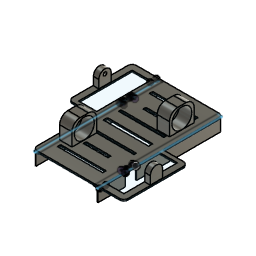
Chassis V4 (Autodesk Fusion 360 design; units mm, degrees)
Autodesk Fusion 360 part; units mm, degrees
note: some values were not read from the file. Set by a fixed rule: which sketch regions a step uses.
sketch "Sketch1" plane through (0, 0, 0) normal (0, 0, 1) x (1, 0, 0)
  line L0 (0, 0) -> (140, 0)
  line L1 (140, 0) -> (140, 150)
  line L2 (140, 150) -> (0, 150)
  line L3 (0, 150) -> (0, 0)
  dimension "d1" = 140
  dimension "d2" = 150
  constraint horizontal L0
  constraint vertical L1
  constraint horizontal L2
  constraint vertical L3
  constraint coincident L0.start L3.end
  measures "d1" distance of L0.start L0.end
  measures "d2" distance of L0.start L2.end
extrude "Extrude1" add sketch "Sketch1" along normal blind 1.75 makes body 1
sketch "Sketch2" plane through (0, 0, 1.75) normal (0, 0, 1) x (-1, 0, 0)
  line L0 (0, -150) -> (0, 0)
  line L1 (0, 0) -> (-140, 0)
  line L2 (-140, 0) -> (-140, -150)
  line L3 (-140, -150) -> (0, -150)
  line L4 (-7.5, -7.5) -> (-132.5, -7.5)
  line L5 (-132.5, -7.5) -> (-132.5, -142.5)
  line L6 (-132.5, -142.5) -> (-7.5, -142.5)
  line L7 (-7.5, -142.5) -> (-7.5, -7.5)
  line L8 (-7.5, -142.5) -> (-29.5, -142.5)
  line L9 (-29.5, -142.5) -> (-29.5, -77.5)
  line L10 (-29.5, -77.5) -> (-7.5, -77.5)
  line L11 (-7.5, -77.5) -> (-7.5, -142.5)
  line L12 (-132.5, -142.5) -> (-132.5, -77.5)
  line L13 (-110.5, -142.5) -> (-132.5, -142.5)
  line L14 (-132.5, -77.5) -> (-110.5, -77.5)
  line L15 (-110.5, -77.5) -> (-110.5, -142.5)
  line L16 (-29.5, -72.5) -> (-29.5, -7.5)
  line L17 (-7.5, -72.5) -> (-29.5, -72.5)
  line L18 (-29.5, -7.5) -> (-7.5, -7.5)
  line L19 (-7.5, -7.5) -> (-7.5, -72.5)
  line L20 (-132.5, -72.5) -> (-132.5, -7.5)
  line L21 (-110.5, -72.5) -> (-132.5, -72.5)
  line L22 (-132.5, -7.5) -> (-110.5, -7.5)
  line L23 (-110.5, -7.5) -> (-110.5, -72.5)
  dimension "d5" = -7.5
  dimension "d6" = 22
  dimension "d7" = 65
  dimension "d10" = -103
  dimension "d11" = 70
  constraint horizontal L8
  constraint vertical L9
  constraint horizontal L10
  constraint vertical L11
  measures "d6" distance of L6.end L8.end
  measures "d7" distance of L6.end L10.end
extrude "Extrude2" cut sketch "Sketch2" against normal up to surface (1.75 mm away) contours L4 L7 L16 L17 L18 L19 | L4 L5 L20 L21 L22 L23 | L6 L7 L8 L9 L10 L11 | L5 L6 L12 L13 L14 L15 bodies 1
sketch "Sketch3" plane through (0, 0, 1.75) normal (0, 0, 1) x (-1, 0, 0)
  line L0 (-110.5, -7.5) -> (-110.5, -72.5)
  line L1 (-132.5, -72.5) -> (-132.5, -7.5)
  line L2 (-132.5, -7.5) -> (-110.5, -7.5)
  line L3 (-110.5, -77.5) -> (-110.5, -142.5)
  line L4 (-110.5, -142.5) -> (-132.5, -142.5)
  line L5 (-132.5, -142.5) -> (-132.5, -77.5)
  line L6 (-132.5, -77.5) -> (-110.5, -77.5)
  line L7 (-7.5, -77.5) -> (-7.5, -142.5)
  line L8 (-7.5, -142.5) -> (-29.5, -142.5)
  line L9 (-29.5, -142.5) -> (-29.5, -77.5)
  line L10 (-29.5, -77.5) -> (-7.5, -77.5)
  line L11 (-7.5, -7.5) -> (-7.5, -72.5)
  line L12 (-29.5, -72.5) -> (-29.5, -7.5)
  line L13 (-29.5, -7.5) -> (-7.5, -7.5)
  line L14 (0, -150) -> (0, 0)
  line L15 (0, 0) -> (-140, 0)
  line L16 (-140, 0) -> (-140, -150)
  line L17 (-140, -150) -> (0, -150)
  line L18 (-29.5, -110) -> (-110.5, -110) construction
  line L19 (-29.5, -40) -> (-110.5, -40) construction
  line L20 (-29.5, -110) -> (-33.25, -110) construction
  line L21 (-30.0705, -117.5) -> (-36.4295, -117.5)
  line L22 (-36.4295, -117.5) -> (-36.4295, -102.5)
  line L23 (-36.4295, -102.5) -> (-30.0705, -102.5)
  line L24 (-30.0705, -102.5) -> (-30.0705, -117.5)
  line L25 (-30.0705, -117.5) -> (-36.4295, -102.5) construction
  line L26 (-36.4295, -117.5) -> (-30.0705, -102.5) construction
  line L27 (-103.5705, -47.5) -> (-109.9295, -47.5)
  line L28 (-103.5705, -32.5) -> (-103.5705, -47.5)
  line L29 (-109.9295, -32.5) -> (-103.5705, -32.5)
  line L30 (-109.9295, -47.5) -> (-109.9295, -32.5)
  line L31 (-110.5, -110) -> (-140, -110) construction
  line L32 (-33.25, -117.5) -> (-33.25, -110) construction
  line L33 (-33.25, -110) -> (-33.25, -102.5) construction
  circle A0 centre (-33.25, -113.75) radius 1.5
  circle A1 centre (-33.25, -106.25) radius 1.5
  line L34 (-106.75, -47.5) -> (-106.75, -40) construction
  line L35 (-106.75, -40) -> (-106.75, -32.5) construction
  circle A2 centre (-106.75, -43.75) radius 1.5
  circle A3 centre (-106.75, -36.25) radius 1.5
  line L36 (-7.5, -110) -> (0, -110) construction
  line L37 (-7.0568, -117.5) -> (-0.4432, -117.5)
  line L38 (-0.4432, -117.5) -> (-0.4432, -102.5)
  line L39 (-0.4432, -102.5) -> (-7.0568, -102.5)
  line L40 (-7.0568, -102.5) -> (-7.0568, -117.5)
  line L41 (-7.0568, -117.5) -> (-0.4432, -102.5) construction
  line L42 (-0.4432, -117.5) -> (-7.0568, -102.5) construction
  line L43 (-139.5568, -47.5) -> (-132.9432, -47.5)
  line L44 (-139.5568, -32.5) -> (-139.5568, -47.5)
  line L45 (-132.9432, -32.5) -> (-139.5568, -32.5)
  line L46 (-132.9432, -47.5) -> (-132.9432, -32.5)
  line L47 (-110.5, -72.5) -> (-132.5, -72.5)
  line L48 (-7.5, -72.5) -> (-29.5, -72.5)
  point P0 (-33.25, -110)
  point P1 (-3.75, -110)
  dimension "d14" = 3.75
  dimension "d15" = 15
  dimension "d18" = -73.5
  dimension "d19" = 70
  dimension "d26" = 3
  dimension "d27" = 3
  dimension "d28" = 3
  dimension "d29" = 3
  dimension "d49" = 15
  dimension "d52" = -132.5
  dimension "d53" = 70
  constraint midpoint L9 L18.start
  constraint midpoint L3 L18.end
  constraint midpoint L12 L19.start
  constraint midpoint L0 L19.end
  constraint perpendicular L9 L20
  constraint horizontal L21
  constraint perpendicular L21 L22
  constraint parallel L21 L23
  constraint parallel L22 L24
  constraint coincident L25 P0
  constraint coincident L26 P0
  constraint coincident P0 L20.end
  constraint coincident L16 L31.end
  constraint perpendicular L16 L31
  constraint midpoint L21 L32.start
  constraint midpoint L23 L33.end
  constraint midpoint L32 A0.centre
  constraint midpoint L33 A1.centre
  constraint midpoint L27 L34.start
  constraint coincident L19 L34.end
  constraint perpendicular L19 L34
  constraint midpoint L29 L35.end
  constraint midpoint L34 A2.centre
  constraint midpoint L35 A3.centre
  constraint midpoint L7 L36.start
  constraint coincident L14 L36.end
  constraint perpendicular L14 L36
  constraint horizontal L37
  constraint perpendicular L37 L38
  constraint parallel L37 L39
  constraint parallel L38 L40
  constraint coincident L41 P1
  constraint coincident L42 P1
  constraint midpoint L36 P1
  measures "d14" distance of L18.start P0
  measures "d15" distance of L21.end L22.end
  measures "d26" diameter of A0
  measures "d27" diameter of A1
  measures "d28" diameter of A2
  measures "d29" diameter of A3
  measures "d49" distance of L37.end L38.end
extrude "Extrude3" add sketch "Sketch3" along normal blind 17.5 contours L37 L38 L39 L40 | L43 L44 L45 L46 bodies 1
extrude "Extrude4" cut sketch "Sketch3" against normal up to surface (1.75 mm away) contours A0 | A1 | A2 | A3 bodies 1
sketch "Sketch4" plane through (132.5, 0, 0) normal (-1, 0, 0) x (0, -1, 0)
  line L0 (-72.5, 0) -> (-7.5, 0)
  line L1 (-7.5, 0) -> (-7.5, 1.75)
  line L2 (-72.5, 1.75) -> (-7.5, 1.75) construction
  line L3 (-40, 1.75) -> (-40, 13.875) construction
  circle A0 centre (-40, 13.875) radius 2.15
  line L4 (-72.5, 1.75) -> (-72.5, 0)
  line L5 (-7.5, 1.75) -> (-72.5, 1.75)
  dimension "d32" = 12.125
  dimension "d33" = 4.3
  constraint midpoint L2 L3.start
  constraint coincident L3.end A0.centre
  measures "d32" distance of L3.start L3.end
  measures "d33" diameter of A0
sketch "Sketch5" plane through (7.5, 0, 0) normal (1, 0, 0) x (0, 1, 0)
  line L0 (77.5, 0) -> (142.5, 0)
  line L1 (142.5, 0) -> (142.5, 1.75)
  line L2 (77.5, 1.75) -> (77.5, 0)
  line L3 (110, 1.75) -> (110, 13.875) construction
  circle A0 centre (110, 13.875) radius 2.15
  line L4 (142.5, 1.75) -> (77.5, 1.75)
  dimension "d34" = 12.125
  dimension "d35" = 4.3
  constraint coincident L3.end A0.centre
  constraint midpoint L3.start L4
  constraint perpendicular L3 L4
  measures "d34" distance of L3.start L3.end
  measures "d35" diameter of A0
extrude "Extrude5" cut sketch "Sketch5" against normal blind 5 contours A0 bodies 1
extrude "Extrude6" cut sketch "Sketch4" against normal blind 5 contours A0 bodies 1
sketch "Sketch6" plane through (0, 0, 1.75) normal (0, 0, 1) x (-1, 0, 0)
  line L0 (-110.4369, -110) -> (-102.9369, -110) construction
  line L1 (-102.9369, -110) -> (-82.9369, -110) construction
  line L2 (-100.4369, -125) -> (-85.4369, -125)
  line L3 (-85.4369, -125) -> (-85.4369, -95)
  line L4 (-85.4369, -95) -> (-100.4369, -95)
  line L5 (-100.4369, -95) -> (-100.4369, -125)
  line L6 (-100.4369, -125) -> (-85.4369, -95) construction
  line L7 (-85.4369, -125) -> (-100.4369, -95) construction
  line L8 (0, 0) -> (-140, 0)
  line L9 (-70, -150) -> (-70, 0) construction
  line L10 (0, -150) -> (0, 0)
  line L11 (-140, 0) -> (-140, -150)
  line L12 (0, -75) -> (-140, -75) construction
  line L13 (-51.9369, -55) -> (-36.9369, -55)
  line L14 (-51.9369, -25) -> (-51.9369, -55)
  line L15 (-36.9369, -25) -> (-51.9369, -25)
  line L16 (-36.9369, -55) -> (-36.9369, -25)
  line L17 (-29.5, -110) -> (-37, -110) construction
  line L18 (-37, -110) -> (-110.4369, -110) construction
  point P0 (-92.9369, -110)
  dimension "d40" = 7.5
  dimension "d41" = 20
  dimension "d42" = 15
  dimension "d43" = 30
  dimension "d46" = 48.5
  dimension "d47" = 70
  dimension "d48" = 7.5
  constraint horizontal L2
  constraint perpendicular L2 L3
  constraint parallel L2 L4
  constraint parallel L3 L5
  constraint coincident L6 P0
  constraint coincident L7 P0
  constraint midpoint L1 P0
  constraint midpoint L8 L9.end
  constraint midpoint L10 L12.start
  constraint midpoint L11 L12.end
  constraint perpendicular L5 L18
  measures "d40" distance of L0.end L0.start
  measures "d41" distance of L0.end L1.end
  measures "d42" distance of L3.end L4.end
  measures "d43" distance of L2.end L3.end
  measures "d48" distance of L17.start L17.end
extrude "Extrude7" add sketch "Sketch6" along normal blind 26 bodies 1
sketch "Sketch7" plane through (51.9369, 0, 0) normal (1, 0, 0) x (0, 1, 0)
  line L0 (25, 1.75) -> (55, 1.75)
  line L1 (55, 1.75) -> (55, 27.75)
  line L2 (55, 27.75) -> (25, 27.75)
  line L3 (25, 27.75) -> (25, 1.75)
  line L4 (40, 1.75) -> (40, 26) construction
  circle A0 centre (40, 13.875) radius 12.125
  dimension "d56" = 24.25
  dimension "d57" = 24.25
  constraint midpoint L0 L4.start
  constraint perpendicular L0 L4
  constraint midpoint L4 A0.centre
  measures "d56" distance of L4.start L4.end
  measures "d57" diameter of A0
sketch "Sketch8" plane through (85.4369, 0, 0) normal (-1, 0, 0) x (0, -1, 0)
  line L0 (-125, 1.75) -> (-95, 1.75)
  line L1 (-95, 1.75) -> (-95, 27.75)
  line L2 (-95, 27.75) -> (-125, 27.75)
  line L3 (-125, 27.75) -> (-125, 1.75)
  line L4 (-110, 1.75) -> (-110, 26) construction
  circle A0 centre (-110, 13.875) radius 12.125
  dimension "d58" = 24.25
  dimension "d59" = 24.25
  constraint midpoint L0 L4.start
  constraint perpendicular L0 L4
  constraint midpoint L4 A0.centre
  measures "d58" distance of L4.start L4.end
  measures "d59" diameter of A0
extrude "Extrude8" cut sketch "Sketch8" against normal up to surface (15 mm away) contours A0 bodies 1
extrude "Extrude9" cut sketch "Sketch7" against normal blind 15 contours A0 bodies 1
fillet "Fillet1" radius 5 4 edges at (0, 0, 0.875) (140, 0, 0.875) (140, 150, 0.875) (0, 150, 0.875) on bodies 1
fillet "Fillet4" radius 10 4 edges at (92.9369, 95, 27.75) (92.9369, 125, 27.75) (44.4369, 55, 27.75) (44.4369, 25, 27.75) on bodies 1
fillet "Fillet5" radius 7.5 4 edges at (136.25, 47.5, 19.25) (136.25, 32.5, 19.25) (3.75, 102.5, 19.25) (3.75, 117.5, 19.25) on bodies 1
sketch "Sketch9" plane through (0, 0, 0) normal (0, 0, -1) x (1, 0, 0)
  circle A0 centre (33.25, -106.25) radius 1.5
  circle A1 centre (106.75, -43.75) radius 1.5
  circle A2 centre (33.25, -113.75) radius 1.5
  circle A3 centre (106.75, -36.25) radius 1.5
  line L0 (110.5, -142.5) -> (110.5, -77.5)
  line L1 (110.5, -77.5) -> (132.5, -77.5)
  line L2 (132.5, -77.5) -> (132.5, -142.5)
  line L3 (132.5, -142.5) -> (110.5, -142.5)
  line L4 (7.5, -72.5) -> (7.5, -7.5)
  line L5 (7.5, -7.5) -> (29.5, -7.5)
  line L6 (29.5, -7.5) -> (29.5, -72.5)
  line L7 (29.5, -72.5) -> (7.5, -72.5)
  line L8 (110.5, -72.5) -> (110.5, -7.5)
  line L9 (110.5, -7.5) -> (132.5, -7.5)
  line L10 (132.5, -7.5) -> (132.5, -72.5)
  line L11 (132.5, -72.5) -> (110.5, -72.5)
  line L12 (7.5, -142.5) -> (7.5, -77.5)
  line L13 (7.5, -77.5) -> (29.5, -77.5)
  line L14 (29.5, -77.5) -> (29.5, -142.5)
  line L15 (29.5, -142.5) -> (7.5, -142.5)
  line L16 (70, 0) -> (70, -150) construction
  line L17 (0, -75) -> (140, -75) construction
  line L18 (0, 0) -> (0, -75) construction
  line L19 (0, 0) -> (0, -75) construction
  line L20 (0, -37.5) -> (140, -37.5) construction
  line L21 (0, -75) -> (0, -145) construction
  line L22 (0, -110) -> (140, -110) construction
  line L23 (85, -35.75) -> (55, -35.75)
  line L24 (55, -35.75) -> (55, -39.25)
  line L25 (55, -39.25) -> (85, -39.25)
  line L26 (85, -39.25) -> (85, -35.75)
  line L27 (85, -35.75) -> (55, -39.25) construction
  line L28 (55, -35.75) -> (85, -39.25) construction
  line L29 (97.5, -72.5) -> (42.5, -72.5)
  line L30 (42.5, -72.5) -> (42.5, -77.5)
  line L31 (42.5, -77.5) -> (97.5, -77.5)
  line L32 (97.5, -77.5) -> (97.5, -72.5)
  line L33 (97.5, -72.5) -> (42.5, -77.5) construction
  line L34 (42.5, -72.5) -> (97.5, -77.5) construction
  line L35 (85, -108.25) -> (55, -108.25)
  line L36 (55, -108.25) -> (55, -111.75)
  line L37 (55, -111.75) -> (85, -111.75)
  line L38 (85, -111.75) -> (85, -108.25)
  line L39 (85, -108.25) -> (55, -111.75) construction
  line L40 (55, -108.25) -> (85, -111.75) construction
  line L41 (0, 0) -> (0, -37.5) construction
  line L42 (0, -37.5) -> (0, -75) construction
  line L43 (0, -75) -> (0, -110) construction
  line L44 (0, -110) -> (0, -151) construction
  line L45 (0, -18.75) -> (140, -18.75) construction
  line L46 (0, -56.25) -> (140, -56.25) construction
  line L47 (0, -92.5) -> (140, -92.5) construction
  line L48 (0, -130.5) -> (140, -130.5) construction
  line L49 (97.5, -54.875) -> (42.5, -54.875)
  line L50 (42.5, -54.875) -> (42.5, -57.625)
  line L51 (42.5, -57.625) -> (97.5, -57.625)
  line L52 (97.5, -57.625) -> (97.5, -54.875)
  line L53 (97.5, -54.875) -> (42.5, -57.625) construction
  line L54 (42.5, -54.875) -> (97.5, -57.625) construction
  line L55 (97.5, -91) -> (42.5, -91)
  line L56 (42.5, -91) -> (42.5, -94)
  line L57 (42.5, -94) -> (97.5, -94)
  line L58 (97.5, -94) -> (97.5, -91)
  line L59 (97.5, -91) -> (42.5, -94) construction
  line L60 (42.5, -91) -> (97.5, -94) construction
  line L61 (97.5, -128.5) -> (42.5, -128.5)
  line L62 (42.5, -128.5) -> (42.5, -132.5)
  line L63 (42.5, -132.5) -> (97.5, -132.5)
  line L64 (97.5, -132.5) -> (97.5, -128.5)
  line L65 (97.5, -128.5) -> (42.5, -132.5) construction
  line L66 (42.5, -128.5) -> (97.5, -132.5) construction
  line L67 (97.5, -16.75) -> (42.5, -16.75)
  line L68 (42.5, -16.75) -> (42.5, -20.75)
  line L69 (42.5, -20.75) -> (97.5, -20.75)
  line L70 (97.5, -20.75) -> (97.5, -16.75)
  line L71 (97.5, -16.75) -> (42.5, -20.75) construction
  line L72 (42.5, -16.75) -> (97.5, -20.75) construction
  line L73 (7.5, -72.5) -> (0, -72.5)
  line L74 (0, -72.5) -> (0, -7.3593)
  line L75 (0, -7.3593) -> (7.5, -7.3593)
  line L76 (7.5, -7.3593) -> (7.5, -72.5)
  line L77 (132.5, -77.5) -> (140, -77.5)
  line L78 (140, -77.5) -> (140, -142.5)
  line L79 (140, -142.5) -> (132.5, -142.5)
  line L80 (132.5, -142.5) -> (132.5, -77.5)
  line L81 (29.5, -7.5) -> (0, -7.5)
  line L82 (0, -7.5) -> (0, 0)
  line L83 (0, 0) -> (29.5, 0)
  line L84 (29.5, 0) -> (29.5, -7.5)
  line L85 (110.5, -142.5) -> (140, -142.5)
  line L86 (140, -142.5) -> (140, -150)
  line L87 (140, -150) -> (110.5, -150)
  line L88 (110.5, -150) -> (110.5, -142.5)
  arc A4 (0, -145) -> (5, -150) centre (5, -145) ccw
  line L89 (5, -150) -> (135, -150)
  arc A5 (135, -150) -> (140, -145) centre (135, -145) ccw
  line L90 (140, -145) -> (140, -5)
  arc A6 (140, -5) -> (135, 0) centre (135, -5) ccw
  line L91 (135, 0) -> (5, 0)
  arc A7 (5, 0) -> (0, -5) centre (5, -5) ccw
  line L92 (0, -5) -> (0, -145)
  point P0 (70, -37.5)
  point P1 (70, -75)
  point P2 (70, -110)
  point P3 (70, -56.25)
  point P4 (70, -92.5)
  point P5 (70, -130.5)
  point P6 (70, -18.75)
  dimension "d74" = 30
  dimension "d75" = 3.5
  dimension "d76" = 55
  dimension "d77" = 5
  dimension "d78" = 30
  dimension "d79" = 3.5
  dimension "d82" = 55
  dimension "d83" = 2.75
  dimension "d84" = 55
  dimension "d85" = 3
  dimension "d86" = 55
  dimension "d87" = 4
  dimension "d88" = 55
  dimension "d89" = 4
  constraint coincident L18.start L19.start
  constraint midpoint L19 L20.start
  constraint midpoint L21 L22.start
  constraint horizontal L23
  constraint perpendicular L23 L24
  constraint parallel L23 L25
  constraint parallel L24 L26
  constraint coincident L27 P0
  constraint coincident L28 P0
  constraint midpoint L20 P0
  constraint horizontal L29
  constraint perpendicular L29 L30
  constraint parallel L29 L31
  constraint parallel L30 L32
  constraint coincident L33 P1
  constraint coincident L34 P1
  constraint midpoint L16 P1
  constraint horizontal L35
  constraint perpendicular L35 L36
  constraint parallel L35 L37
  constraint parallel L36 L38
  constraint coincident L39 P2
  constraint coincident L40 P2
  constraint midpoint L22 P2
  constraint midpoint L41 L45.start
  constraint midpoint L42 L46.start
  constraint midpoint L43 L47.start
  constraint midpoint L44 L48.start
  constraint horizontal L49
  constraint perpendicular L49 L50
  constraint parallel L49 L51
  constraint parallel L50 L52
  constraint coincident L53 P3
  constraint coincident L54 P3
  constraint midpoint L46 P3
  constraint horizontal L55
  constraint perpendicular L55 L56
  constraint parallel L55 L57
  constraint parallel L56 L58
  constraint coincident L59 P4
  constraint coincident L60 P4
  constraint midpoint L47 P4
  constraint horizontal L61
  constraint perpendicular L61 L62
  constraint parallel L61 L63
  constraint parallel L62 L64
  constraint coincident L65 P5
  constraint coincident L66 P5
  constraint midpoint L48 P5
  constraint horizontal L67
  constraint perpendicular L67 L68
  constraint parallel L67 L69
  constraint parallel L68 L70
  constraint coincident L71 P6
  constraint coincident L72 P6
  constraint midpoint L45 P6
  constraint horizontal L73
  constraint vertical L74
  constraint horizontal L75
  constraint vertical L76
  constraint coincident L41 L74.end
  constraint coincident L4.start L7.end
  constraint horizontal L77
  constraint vertical L78
  constraint horizontal L79
  constraint vertical L80
  constraint coincident L1.end L2.start
  constraint horizontal L81
  constraint vertical L82
  constraint horizontal L83
  constraint vertical L84
  constraint coincident L5.end L6.start
  constraint horizontal L85
  constraint vertical L86
  constraint horizontal L87
  constraint vertical L88
  constraint coincident L0.start L3.end
  measures "d74" distance of L24.end L25.end
  measures "d75" distance of L23.end L24.end
  measures "d76" distance of L30.end L31.end
  measures "d77" distance of L29.end L30.end
  measures "d78" distance of L36.end L37.end
  measures "d79" distance of L35.end L36.end
  measures "d82" distance of L50.end L51.end
  measures "d83" distance of L49.end L50.end
  measures "d84" distance of L56.end L57.end
  measures "d85" distance of L55.end L56.end
  measures "d86" distance of L62.end L63.end
  measures "d87" distance of L61.end L62.end
  measures "d88" distance of L68.end L69.end
  measures "d89" distance of L67.end L68.end
extrude "Extrude10" cut sketch "Sketch9" against normal up to surface (1.75 mm away) contours L23 L24 L25 L26 | L29 L30 L31 L32 | L35 L36 L37 L38 | L49 L50 L51 L52 | L55 L56 L57 L58 | L61 L62 L63 L64 | L67 L68 L69 L70 bodies 1
extrude "Extrude11" cut sketch "Sketch9" against normal up to surface (1.75 mm away) contours L3 L79 L85 L86 L87 L88 L89 A5 L90 | L2 L77 L78 L79 L80 L85 L90 | L4 L73 L74 L76 L81 L92 | L74 L75 L76 L81 L82 L92 | L5 L75 L76 L81 L82 L83 L84 L91 A7 L92 bodies 1
fillet "Fillet6" radius 5 4 edges at (140, 77.5, 0.875) (110.5, 150, 0.875) (29.5, 0, 0.875) (0, 72.5, 0.875) on bodies 1
sketch "Sketch10" plane through (0, 0, 0) normal (0, 0, -1) x (1, 0, 0)
  arc A0 (5, -72.5) -> (0, -77.5) centre (5, -77.5) ccw
  line L0 (0, -77.5) -> (0, -145)
  arc A1 (0, -145) -> (5, -150) centre (5, -145) ccw
  line L1 (5, -150) -> (105.5, -150)
  arc A2 (105.5, -150) -> (110.5, -145) centre (105.5, -145) ccw
  line L2 (110.5, -145) -> (110.5, -77.5)
  line L3 (110.5, -77.5) -> (135, -77.5)
  arc A3 (135, -77.5) -> (140, -72.5) centre (135, -72.5) ccw
  line L4 (140, -72.5) -> (140, -5)
  arc A4 (140, -5) -> (135, 0) centre (135, -5) ccw
  line L5 (135, 0) -> (34.5, 0)
  arc A5 (34.5, 0) -> (29.5, -5) centre (34.5, -5) ccw
  line L6 (29.5, -5) -> (29.5, -72.5)
  line L7 (29.5, -72.5) -> (5, -72.5)
  line L8 (7.5, -142.5) -> (7.5, -77.5)
  line L9 (7.5, -77.5) -> (29.5, -77.5)
  line L10 (29.5, -77.5) -> (29.5, -142.5)
  line L11 (29.5, -142.5) -> (7.5, -142.5)
  line L12 (110.5, -72.5) -> (110.5, -7.5)
  line L13 (110.5, -7.5) -> (132.5, -7.5)
  line L14 (132.5, -7.5) -> (132.5, -72.5)
  line L15 (132.5, -72.5) -> (110.5, -72.5)
  circle A6 centre (106.75, -36.25) radius 1.5
  circle A7 centre (33.25, -113.75) radius 1.5
  circle A8 centre (106.75, -43.75) radius 1.5
  circle A9 centre (33.25, -106.25) radius 1.5
  line L16 (97.5, -132.5) -> (42.5, -132.5)
  line L17 (42.5, -132.5) -> (42.5, -128.5)
  line L18 (42.5, -128.5) -> (97.5, -128.5)
  line L19 (97.5, -128.5) -> (97.5, -132.5)
  line L20 (85, -111.75) -> (55, -111.75)
  line L21 (55, -111.75) -> (55, -108.25)
  line L22 (55, -108.25) -> (85, -108.25)
  line L23 (85, -108.25) -> (85, -111.75)
  line L24 (97.5, -77.5) -> (42.5, -77.5)
  line L25 (42.5, -77.5) -> (42.5, -72.5)
  line L26 (42.5, -72.5) -> (97.5, -72.5)
  line L27 (97.5, -72.5) -> (97.5, -77.5)
  line L28 (97.5, -94) -> (42.5, -94)
  line L29 (42.5, -94) -> (42.5, -91)
  line L30 (42.5, -91) -> (97.5, -91)
  line L31 (97.5, -91) -> (97.5, -94)
  line L32 (97.5, -20.75) -> (42.5, -20.75)
  line L33 (42.5, -20.75) -> (42.5, -16.75)
  line L34 (42.5, -16.75) -> (97.5, -16.75)
  line L35 (97.5, -16.75) -> (97.5, -20.75)
  line L36 (85, -39.25) -> (55, -39.25)
  line L37 (55, -39.25) -> (55, -35.75)
  line L38 (55, -35.75) -> (85, -35.75)
  line L39 (85, -35.75) -> (85, -39.25)
  line L40 (97.5, -57.625) -> (42.5, -57.625)
  line L41 (42.5, -57.625) -> (42.5, -54.875)
  line L42 (42.5, -54.875) -> (97.5, -54.875)
  line L43 (97.5, -54.875) -> (97.5, -57.625)
  line L44 (110.5, -7.5) -> (110.5, 0) construction
  line L45 (29.5, -142.5) -> (29.5, -150) construction
  line L46 (29.5, -150) -> (31.5, -150) construction
  line L47 (31.5, -150) -> (36.5, -150)
  line L48 (36.5, -150) -> (36.5, 0)
  line L49 (36.5, 0) -> (31.5, 0)
  line L50 (31.5, 0) -> (31.5, -150)
  line L51 (110.5, 0) -> (108.5, 0) construction
  line L52 (108.5, 0) -> (103.5, 0)
  line L53 (103.5, 0) -> (103.5, -150)
  line L54 (103.5, -150) -> (108.5, -150)
  line L55 (108.5, -150) -> (108.5, 0)
  circle A10 centre (33.25, -113.75) radius 1.75
  circle A11 centre (33.25, -106.25) radius 1.75
  circle A12 centre (106.75, -36.25) radius 1.75
  circle A13 centre (106.75, -43.75) radius 1.75
  line L56 (33.25, -113.75) -> (33.25, -116.75)
  line L57 (33.25, -106.25) -> (33.25, -103.25)
  line L58 (36.5, -103.25) -> (31.5, -103.25)
  line L59 (36.5, -116.75) -> (31.5, -116.75)
  line L60 (106.75, -36.25) -> (106.75, -33.25)
  line L61 (106.75, -43.75) -> (106.75, -46.75)
  line L62 (103.5, -46.75) -> (108.5, -46.75)
  line L63 (103.5, -33.25) -> (108.5, -33.25)
  dimension "d94" = 2
  dimension "d95" = 5
  dimension "d96" = 2
  dimension "d97" = 5
  dimension "d98" = 3.5
  dimension "d99" = 3.5
  dimension "d100" = 3.5
  dimension "d101" = 3.5
  dimension "d108" = 3
  dimension "d109" = 3
  dimension "d110" = 3
  dimension "d111" = 3
  constraint coincident L12.end L13.start
  constraint coincident L5 L44.end
  constraint perpendicular L5 L44
  constraint coincident L10.end L11.start
  constraint coincident L1 L45.end
  constraint perpendicular L1 L45
  constraint perpendicular L45 L46
  constraint horizontal L47
  constraint vertical L48
  constraint horizontal L49
  constraint vertical L50
  constraint perpendicular L44 L51
  constraint horizontal L52
  constraint vertical L53
  constraint horizontal L54
  constraint vertical L55
  constraint concentric A7 A10
  constraint concentric A9 A11
  constraint concentric A6 A12
  constraint concentric A8 A13
  constraint coincident A7.centre A10.centre
  constraint parallel L48 L56
  constraint coincident A9.centre A11.centre
  constraint vertical L57
  constraint coincident L48 L58.start
  constraint coincident L50 L58.end
  constraint perpendicular L50 L58
  constraint coincident L48 L59.start
  constraint coincident L50 L59.end
  constraint perpendicular L50 L59
  constraint coincident A6.centre A12.centre
  constraint vertical L60
  constraint coincident A8.centre A13.centre
  constraint vertical L61
  constraint coincident L53 L62.start
  constraint coincident L55 L62.end
  constraint perpendicular L55 L62
  constraint coincident L53 L63.start
  constraint coincident L55 L63.end
  constraint perpendicular L55 L63
  measures "d94" distance of L45.end L46.end
  measures "d95" distance of L46.end L47.end
  measures "d96" distance of L44.end L51.end
  measures "d97" distance of L51.end L52.end
  measures "d98" diameter of A10
  measures "d99" diameter of A11
  measures "d100" diameter of A12
  measures "d101" diameter of A13
  measures "d108" distance of A7.centre L56.end
  measures "d109" distance of A9.centre L57.end
  measures "d110" distance of A6.centre L60.end
  measures "d111" distance of A8.centre L61.end
extrude "Extrude12" add sketch "Sketch10" along normal blind 1 separate body contours L5 A5 L48 L49 L50 L58 | L1 L47 L48 L50 L59 | L1 A2 L53 L54 L55 L62 | L5 L52 L53 L55 L63 makes body 2 at (34.8333, 34.75, 0) makes body 3 at (105.1667, 115.25, 0) makes body 4 at (33.1667, 127.8333, 0) makes body 5 at (105.1667, 11.0833, 0)
sketch "Sketch11" plane through (0, 0, -1) normal (0, 0, -1) x (1, 0, 0)
  line L0 (103.5, -46.75) -> (103.5, -150)
  line L1 (103.5, -150) -> (105.5, -150)
  arc A0 (105.5, -150) -> (108.5, -149) centre (105.5, -145) ccw
  line L2 (108.5, -149) -> (108.5, -46.75)
  line L3 (108.5, 0) -> (107.5, 0)
  line L4 (107.5, 0) -> (107.5, -150)
  line L5 (107.5, -150) -> (108.5, -150)
  line L6 (108.5, -150) -> (108.5, 0)
  line L7 (108.5, -46.75) -> (103.5, -46.75)
  line L8 (103.5, -46.75) -> (108.5, -46.75)
  line L9 (108.5, -33.25) -> (103.5, -33.25)
  line L10 (108.5, -46.75) -> (107.5, -46.75)
  line L11 (108.5, -33.25) -> (107.5, -33.25)
  point P0 (108.5, -33.25)
  point P1 (103.5, -33.25)
  dimension "d104" = 1
  constraint horizontal L3
  constraint vertical L4
  constraint horizontal L5
  constraint vertical L6
  constraint coincident L0.start L7.end
  constraint coincident L2.end L7.start
  constraint coincident P0 L9.start
  constraint coincident P1 L9.end
  constraint coincident L4 L10.end
  constraint coincident L7 L10.end
  constraint coincident L4 L11.end
  constraint coincident L9 L11.end
  measures "d104" distance of L3.start L3.end
sketch "Sketch12" plane through (0, 0, -1) normal (0, 0, -1) x (1, 0, 0)
  line L0 (36.5, -103.25) -> (36.5, 0)
  line L1 (36.5, 0) -> (34.5, 0)
  arc A0 (34.5, 0) -> (31.5, -1) centre (34.5, -5) ccw
  line L2 (31.5, -1) -> (31.5, -103.25)
  line L3 (31.5, -150) -> (32.5, -150)
  line L4 (32.5, -150) -> (32.5, 0)
  line L5 (32.5, 0) -> (31.5, 0)
  line L6 (31.5, 0) -> (31.5, -150)
  line L7 (31.5, -103.25) -> (36.5, -103.25)
  line L8 (31.5, -116.75) -> (36.5, -116.75)
  line L9 (31.5, -103.25) -> (36.5, -103.25)
  point P0 (31.5, -116.75)
  point P1 (36.5, -116.75)
  dimension "d105" = 1
  constraint horizontal L3
  constraint vertical L4
  constraint horizontal L5
  constraint vertical L6
  constraint coincident P0 L8.start
  constraint coincident P1 L8.end
  constraint coincident L2.end L7.start
  constraint coincident L0.start L7.end
  measures "d105" distance of L3.start L3.end
extrude "Extrude14" add sketch "Sketch12" sketch "Sketch11" along normal blind 15 contours A0 L2 L4 L6 L7 L9 | L3 L4 L6 L8 of sketch 2 contours A0 L2 L4 L6 L7 L8 L10 | L3 L4 L6 L9 L11 bodies 4 5 2 3
